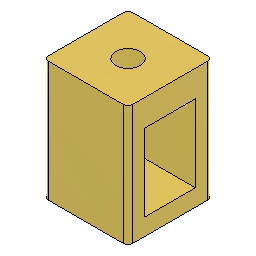
Desk Mount (Autodesk Fusion 360 design; units mm, degrees)
Autodesk Fusion 360 part; units mm, degrees
sketch "Sketch1" plane through (0, 0, 0) normal (0, 1, 0) x (1, 0, 0)
  line L0 (-17.5, 17.5) -> (17.5, 17.5)
  line L1 (17.5, 17.5) -> (17.5, -17.5)
  line L2 (17.5, -17.5) -> (-17.5, -17.5)
  line L3 (-17.5, -17.5) -> (-17.5, 17.5)
  line L4 (-17.5, 17.5) -> (17.5, -17.5) construction
  line L5 (17.5, 17.5) -> (-17.5, -17.5) construction
  dimension "d1" = 35
  dimension "d2" = 35
  constraint horizontal L0
  constraint perpendicular L0 L1
  constraint parallel L0 L2
  constraint parallel L1 L3
  constraint coincident L4 origin
  constraint coincident L5 origin
  measures "d1" distance of L1.end L2.end
  measures "d2" distance of L0.end L1.end
extrude "Extrude1" add sketch "Sketch1" along normal blind 50 makes body 1
sketch "Sketch2" plane through (0, 50, 0) normal (0, 1, 0) x (-1, 0, 0)
  line L0 (17.5, 17.5) -> (-17.5, 17.5)
  line L1 (-17.5, 17.5) -> (-17.5, -17.5)
  line L2 (-17.5, -17.5) -> (17.5, -17.5)
  line L3 (17.5, -17.5) -> (17.5, 17.5)
  circle A0 centre (0, 0) radius 5.05
  dimension "d5" = 10.1
  constraint coincident A0.centre origin
  measures "d5" diameter of A0
extrude "Extrude2" cut sketch "Sketch2" against normal blind 20 contours A0 bodies 1
sketch "Sketch3" plane through (17.5, 0, 0) normal (1, 0, 0) x (0, 0, -1)
  line L0 (-17.5, 0) -> (17.5, 0)
  line L1 (17.5, 0) -> (17.5, 50)
  line L2 (17.5, 50) -> (-17.5, 50)
  line L3 (-17.5, 50) -> (-17.5, 0)
  line L4 (-10.5, 7) -> (10.5, 7)
  line L5 (10.5, 7) -> (10.5, 43)
  line L6 (10.5, 43) -> (-10.5, 43)
  line L7 (-10.5, 43) -> (-10.5, 7)
  line L8 (-5.05, 30) -> (5.05, 30)
  line L9 (-10.5, 7) -> (-10.5, 19) construction
  line L10 (-10.5, 19) -> (10.5, 19)
  dimension "d8" = -7
  dimension "d10" = 12
  constraint perpendicular L4 L9
  constraint coincident L5 L10.end
  constraint perpendicular L5 L10
  measures "d10" distance of L4.start L9.end
extrude "Extrude3" cut sketch "Sketch3" against normal blind 20 contours L4 L5 L7 L10 bodies 1
draft "Draft1" angle 45 neutral plane through (-2.5, 0, 0) pull (1, 0, 0) 1 faces at (10.8333, 19, 3.5) on bodies 1
fillet "Fillet2" radius 2 4 edges at (-17.5, 25, 17.5) (17.5, 25, 17.5) (17.5, 25, -17.5) (-17.5, 25, -17.5) on bodies 1
delete_face "DeleteFace2" 1 faces at (-2.5, 15, -3.5) on bodies 1
copy_body "Body->Comp1" bodies 1 removing the originals makes body 2 in component "Desk Mount"
component "Desk Mount" placed x (1, 0, 0) y (0, 1, 0) z (0, 0, 1) at (0, 0, 0)
named bodies: "Desk Mount"
